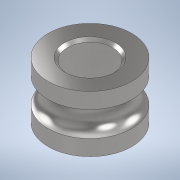
# Autodesk Inventor part: 6138k63_race_inner
Saved by Autodesk Inventor 2020.1 (Build 241239000, 239)
## iProperties
Created: 2019-10-27
Part Number: 6138k63_race_inner
Material: Stainless Steel, 440C
Document SubType Name: Modeling
Designer: agmle
Mass: 0.470458 g
Surface Area: 1.53453 cm^2
Volume: 0.0607043 cm^3
Density: 7.75 g/cm^3
Appearance: Semi-Polished
Author: agmle
Autodesk Inventor part; units mm, degrees
ref_plane "YZ Plane" through (0, 0, 0) normal (1, 0, 0) x (0, 1, 0)
ref_plane "XZ Plane" through (0, 0, 0) normal (0, 1, 0) x (-1, 0, 0)
ref_plane "XY Plane" through (0, 0, 0) normal (0, 0, 1) x (1, 0, 0)
sketch "Sketch1" plane through (0, 0, 0) normal (0, 0, 1) x (1, 0, 0)
  line L0 (0, 0) -> (1.5875, 0) construction
  line L1 (1.5875, 0) -> (1.5875, 1.7859)
  line L2 (1.5875, 1.7859) -> (1.7859, 1.9844)
  line L3 (1.7859, 1.9844) -> (2.9308, 1.9844)
  line L4 (2.9308, 1.9844) -> (2.9308, 1.8852)
  line L5 (2.9308, 1.8852) -> (2.9308, 1.8852)
  line L6 (2.9308, 1.8852) -> (2.9308, 0.9151)
  line L7 (2.9308, 0.9151) -> (2.9308, 0.9151)
  line L8 (2.9308, 0.9151) -> (2.9308, 0.8819)
  line L9 (1.5875, 0) -> (4.5549, 0) construction
  arc A0 (2.9308, 0.8819) -> (2.2599, 0) centre (3.175, 0) ccw
  line L10 (1.5875, 0) -> (1.5875, -1.7859)
  line L11 (1.5875, -1.7859) -> (1.7859, -1.9844)
  line L12 (1.7859, -1.9844) -> (2.9308, -1.9844)
  line L13 (2.9308, -1.9844) -> (2.9308, -1.8852)
  line L14 (2.9308, -1.8852) -> (2.9308, -0.9151)
  line L15 (2.9308, -0.9151) -> (2.9308, -0.8819)
  arc A1 (2.2599, 0) -> (2.9308, -0.8819) centre (3.175, 0) ccw
  line L16 (0, -2.7781) -> (0, 2.7781) projected
  dimension "d1" = 1.9844
  dimension "d2" = 2.9308
  dimension "d3" = 1.5875
  dimension "d4" = 0.2806
  dimension "d5" = 1.1448
  dimension "d6" = 0.97
  dimension "d7" = 0.0992
  dimension "d8" = 0
  dimension "d9" = 0.9151
  dimension "d10" = 0.2442
  constraints: 32 end point, 8 symmetric about line, 6 point on line, 5 perpendicular, 4 point on circle, 2 centre point, 2 horizontal, 1 parallel, 1 other
  measures "d1" distance between parallel lines of L0 L3
  measures "d2" distance from line of L0.start L4
  measures "d3" distance from line of L0.start L1
  measures "d4" distance of L1.end L2.end
  measures "d5" distance of L2.end L3.end
  measures "d6" distance of L5.end L6.end
  measures "d7" distance between parallel lines of L3 L5
  measures "d8" distance between parallel lines of L4 L6
  measures "d9" radius of A0
  measures "d10" distance from line of L8 A0.centre
revolve "Revolution1" add sketch "Sketch1" angle 360 about axis through (0, -10, 0) along (0, 1, 0)
body "Solid1"
